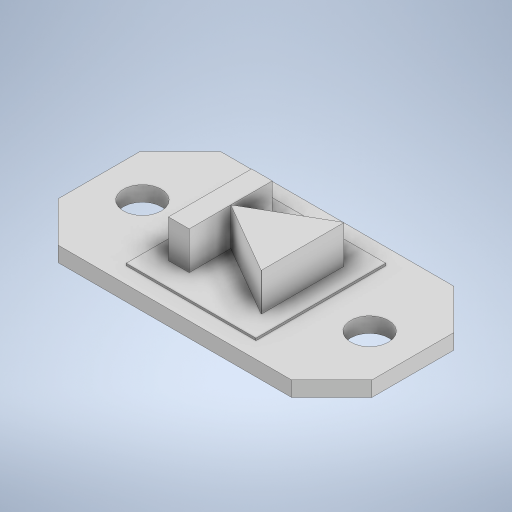
# Autodesk Inventor part: guzik
Saved by Autodesk Inventor 2024.3 (Build 283343000, 343)
## iProperties
Created: 2025-07-27
Part Number: guzik
Material: Ogólny
Document SubType Name: Modeling
Designer: User
Density: 1 g/cm^3
Appearance: Domyślna
Author: User
Autodesk Inventor part; units mm, degrees
ref_plane "YZ Plane" through (0, 0, 0) normal (1, 0, 0) x (0, 1, 0)
ref_plane "XZ Plane" through (0, 0, 0) normal (0, 1, 0) x (-1, 0, 0)
ref_plane "XY Plane" through (0, 0, 0) normal (0, 0, 1) x (1, 0, 0)
sketch "Szkic1" plane through (0, 0, 0) normal (0, 1, 0) x (-1, 0, 0)
  line L0 (-15, 8) -> (15, 8)
  line L1 (15, 8) -> (15, -8)
  line L2 (15, -8) -> (-15, -8)
  line L3 (-15, -8) -> (-15, 8)
  line L4 (-15, 8) -> (15, -8) construction
  line L5 (15, 8) -> (-15, -8) construction
  line L6 (-6, 6) -> (6, 6)
  line L7 (6, 6) -> (6, -6)
  line L8 (6, -6) -> (-6, -6)
  line L9 (-6, -6) -> (-6, 6)
  line L10 (-6, 6) -> (6, -6) construction
  line L11 (6, 6) -> (-6, -6) construction
  circle A0 centre (0, 0) radius 1.75
  dimension "d0" = 30
  dimension "d1" = 16
  dimension "d2" = 12
  dimension "d3" = 12
  dimension "d4" = 3.5
  constraints: 24 end point, 4 midpoint, 4 parallel, 2 horizontal, 2 perpendicular, 1 centre point, 1 coincident
  measures "d0" distance of L1.end L2.end
  measures "d1" distance of L0.end L1.end
  measures "d2" distance of L7.end L8.end
  measures "d3" distance of L6.end L7.end
  measures "d4" diameter of A0
extrude "Wyciągnięcie proste1" add sketch "Szkic1" along normal blind 1.4 contours L0 L1 L2 L3 | L6 L7 L8 L9 | A0
extrude "Wyciągnięcie proste2" add sketch "Szkic1" along normal blind 1.6 contours L6 L7 L8 L9 | A0
extrude "Wyciągnięcie proste3" cut sketch "Szkic1" along normal blind 1 contours A0
chamfer "Faza1" distance 4 angle 45 4 edges at (15, 0.7, 8) (15, 0.7, -8) (-15, 0.7, 8) (-15, 0.7, -8)
offset faces "Rozmiar1" outward -0.5 faces at (-3.6667, 0.4667, 8) (-12.3333, 0.4667, 6.6667) (12.3333, 0.4667, 6.6667) (15, 0.4667, 1.3333) (13.6667, 0.4667, -5.3333) (3.6667, 0.4667, -8) (-13.6667, 0.4667, -5.3333) (-15, 0.4667, -1.3333)
sketch "Szkic2" plane through (0, 1.4, 0) normal (0, 1, 0) x (1, 0, 0)
  line L0 (-6, -6) -> (6, -6) projected
  line L1 (-6, 6) -> (6, 6) projected
  line L2 (-6, -6) -> (6, -6)
  line L3 (6, -6) -> (6, 6)
  line L4 (6, 6) -> (-6, 6)
  line L5 (-6, 6) -> (-6, -6)
  line L6 (0, 0) -> (-10.5, 0)
  line L7 (-10.5, 0) -> (10.5, 0)
  circle A0 centre (10.5, 0) radius 1.75
  circle A1 centre (-10.5, 0) radius 1.75
  dimension "d16" = 10.5
  dimension "d17" = 21
  dimension "d18" = 3.5
  dimension "d19" = 3.5
  constraints: 12 end point, 2 centre point, 2 coincident, 2 horizontal, 2 parallel, 1 perpendicular, 1 point on line
  measures "d16" distance of L6.start L6.end
  measures "d17" distance of L6.end L7.end
  measures "d18" diameter of A0
  measures "d19" diameter of A1
extrude "Wyciągnięcie proste4" cut sketch "Szkic2" against normal blind 10 contours A0 | A1
sketch "Szkic4" plane through (0, 1.6, 0) normal (0, 1, 0) x (1, 0, 0)
  line L0 (-4.2511, -3.84) -> (-4.2511, 0)
  line L1 (5.76, 0) -> (4.32, 0)
  line L2 (-2.3311, 0) -> (-2.3311, 3.84)
  line L3 (4.32, 0) -> (4.32, 3.84)
  line L4 (0, -5.76) -> (0, 5.76)
  line L5 (0, 5.76) -> (0, -5.76)
  line L6 (5.76, -5.76) -> (-5.76, -5.76)
  line L7 (-5.76, -5.76) -> (5.76, -5.76)
  line L8 (4.32, 3.84) -> (-2.3311, 0)
  line L9 (5.76, -5.76) -> (5.76, 5.76)
  line L10 (5.76, 5.76) -> (5.76, -5.76)
  line L11 (5.76, 0) -> (-5.76, 0)
  line L12 (5.76, 5.76) -> (-5.76, 5.76)
  line L13 (-5.76, 5.76) -> (5.76, 5.76)
  line L14 (5.76, 5.76) -> (-5.76, 5.76)
  circle A0 centre (0, 0) radius 5.76
  line L15 (-5.76, -5.76) -> (-5.76, 5.76)
  line L16 (-5.76, 5.76) -> (-5.76, -5.76)
  line L17 (-5.76, 5.76) -> (-5.76, -5.76)
  line L18 (4.32, 0) -> (4.32, -3.84)
  line L19 (4.32, -3.84) -> (-2.3311, 0)
  line L20 (-2.3311, 0) -> (-2.3311, -3.84)
  line L21 (-4.2511, 3.84) -> (-4.2511, 0)
  line L22 (-2.3311, -3.84) -> (-4.2511, -3.84)
  line L23 (-2.3311, 3.84) -> (-4.2511, 3.84)
  line L24 (6, -6) -> (-6, -6) projected
  line L25 (6, 6) -> (-6, 6) projected
  line L26 (5.76, -5.76) -> (-5.76, -5.76)
  line L27 (-5.76, -5.76) -> (-5.76, 5.76)
  line L28 (-5.76, 5.76) -> (5.76, 5.76)
  line L29 (5.76, 5.76) -> (5.76, -5.76)
  point P0 (-16.6045, -17.9068)
  point P1 (5.76, -5.76)
  point P2 (-5.76, -5.76)
  point P3 (4.32, 3.8099)
  point P4 (4.3023, 3.8298)
  point P5 (4.3023, -3.8298)
  point P6 (4.32, -3.8099)
  constraints: 56 end point, 13 parallel, 4 midpoint, 4 point on circle, 3 point on line, 2 tangent, 1 centre point, 1 horizontal, 1 perpendicular
extrude "Wyciągnięcie proste5" add sketch "Szkic4" along normal blind 3.5 contours L0 L11 L20 L22 | L21 L23 L2 L11 | L8 L4 L11 | L11 L4 L19 | L8 A0 L3 L11 L4 | L11 L18 A0 L19 L4
move faces "Przesuń1" translate (0, -1.75, 0) faces at (-0.0229, 1, 0.3868)
